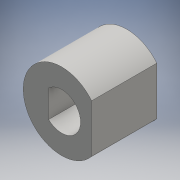
# Autodesk Inventor part: shaft-adapter
Saved by Autodesk Inventor 2016 (Build 200138000, 138)
## iProperties
Created: 2016-10-30
Part Number: shaft-adapter
Material: Generic
Document SubType Name: Modeling
Designer: Matt Ruffner
Density: 1 g/cm^3
Appearance: Default
Author: Matt Ruffner
Autodesk Inventor part; units mm, degrees
ref_plane "YZ Plane" through (0, 0, 0) normal (1, 0, 0) x (0, 1, 0)
ref_plane "XZ Plane" through (0, 0, 0) normal (0, 1, 0) x (-1, 0, 0)
ref_plane "XY Plane" through (0, 0, 0) normal (0, 0, 1) x (1, 0, 0)
sketch "Sketch1" plane through (0, 0, 0) normal (0, 1, 0) x (-1, 0, 0)
  arc A0 (-2.1, -2.0718) -> (-2.1, 2.0718) centre (0, 0) ccw
  arc A1 (1, 1.05) -> (1, -1.05) centre (0, 0) ccw
  line L0 (1, 0) -> (1, 1.05)
  line L1 (1, 0) -> (1, -1.05)
  arc A2 (-2.2177, -1.9454) -> (-2.2177, 1.9454) centre (0, 0) ccw
  line L2 (-2.3, -1.8473) -> (-2.3, 1.8473)
  arc A3 (-2.3, -1.8473) -> (-2.3, 1.8473) centre (0, 0) ccw
  dimension "d0" = 5.9
  dimension "d1" = 2.9
  dimension "d2" = 1
  dimension "d7" = 2.3
  constraints: 8 point on circle, 6 end point, 4 centre point, 4 coincident, 2 vertical, 1 point on line
  measures "d0" diameter of A0
  measures "d1" diameter of A1
  measures "d2" distance of A1.centre L0.start
  measures "d7" distance from line of L2 point (0, 0)
extrude "Extrusion1" add sketch "Sketch1" along normal blind 5
body "Solid1"
